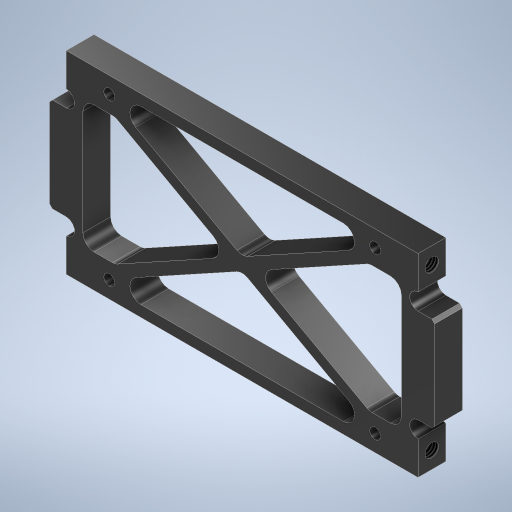
# Autodesk Inventor part: LegLinkBraceFrame
Saved by Autodesk Inventor 2024.2 (Build 282272000, 272)
## iProperties
Created: 2024-01-05
Part Number: LegLinkBraceFrame
Material: Aluminum 7075
Document SubType Name: Modeling
Designer: Masato Kubotera
Density: 2.81 g/cm^3
Appearance: Glossy - Black
Mass: 11.6625 g
Surface Area: 47.7408 cm^2
Volume: 4.15035 cm^3
Vendor: meviy
Author: Masato Kubotera
Autodesk Inventor part; units mm, degrees
ref_plane "YZ Plane" through (0, 0, 0) normal (1, 0, 0) x (0, 1, 0)
ref_plane "XZ Plane" through (0, 0, 0) normal (0, 1, 0) x (-1, 0, 0)
ref_plane "XY Plane" through (0, 0, 0) normal (0, 0, 1) x (1, 0, 0)
sketch "Sketch1" plane through (0, 0, 0) normal (1, 0, 0) x (0, 1, 0)
  line L0 (-31.75, 17.5) -> (31.75, 17.5)
  line L1 (31.75, 17.5) -> (31.75, -17.5)
  line L2 (31.75, -17.5) -> (-31.75, -17.5)
  line L3 (-31.75, -17.5) -> (-31.75, 17.5)
  line L4 (-31.75, 17.5) -> (31.75, -17.5) construction
  line L5 (31.75, 17.5) -> (-31.75, -17.5) construction
  line L6 (0, 17.5) -> (0, -17.5)
  line L7 (-31.75, 0) -> (31.75, 0) construction
  line L8 (31.75, 8.5) -> (34.75, 8.5)
  line L9 (34.75, 8.5) -> (34.75, -8.5)
  line L10 (34.75, -8.5) -> (31.75, -8.5)
  arc A0 (31.75, 11.5) -> (31.75, 8.5) centre (31.75, 10) ccw
  arc A1 (31.75, -8.5) -> (31.75, -11.5) centre (31.75, -10) ccw
  line L11 (31.75, 14.5) -> (25.75, 14.5) construction
  line L12 (26.75, 11.5) -> (23.4506, 11.5)
  line L13 (22.4852, 11.2516) -> (5.2495, 1.7516)
  line L14 (28.75, 9.5) -> (28.75, -9.5)
  line L15 (20.278, 13.5) -> (20.278, 13.5)
  line L16 (19.2434, 11.7484) -> (0.9654, 1.674)
  line L17 (18.278, 15.5) -> (-18.278, 15.5)
  line L18 (-20.278, 13.5) -> (-20.278, 13.5)
  line L19 (-19.2434, 11.7484) -> (-0.9654, 1.674)
  line L20 (26.75, -11.5) -> (23.4506, -11.5)
  line L21 (22.4852, -11.2516) -> (5.2495, -1.7516)
  arc A2 (20.278, 13.5) -> (18.278, 15.5) centre (18.278, 13.5) ccw
  arc A3 (19.2434, 11.7484) -> (20.278, 13.5) centre (18.278, 13.5) ccw
  arc A4 (-18.278, 15.5) -> (-20.278, 13.5) centre (-18.278, 13.5) ccw
  arc A5 (-20.278, 13.5) -> (-19.2434, 11.7484) centre (-18.278, 13.5) ccw
  arc A6 (-0.9654, 1.674) -> (0.9654, 1.674) centre (0, 3.4255) ccw
  arc A7 (23.4506, 11.5) -> (22.4852, 11.2516) centre (23.4506, 9.5) ccw
  arc A8 (28.75, 9.5) -> (26.75, 11.5) centre (26.75, 9.5) ccw
  arc A9 (26.75, -11.5) -> (28.75, -9.5) centre (26.75, -9.5) ccw
  arc A10 (22.4852, -11.2516) -> (23.4506, -11.5) centre (23.4506, -9.5) ccw
  arc A11 (5.2495, 1.7516) -> (5.2495, -1.7516) centre (6.2149, 0) ccw
  line L22 (25.75, 16) -> (25.75, 13) construction
  line L23 (19.2434, -11.7484) -> (0.9654, -1.674)
  line L24 (18.278, -15.5) -> (-18.278, -15.5)
  line L25 (-19.2434, -11.7484) -> (-0.9654, -1.674)
  arc A12 (18.278, -15.5) -> (20.278, -13.5) centre (18.278, -13.5) ccw
  arc A13 (20.278, -13.5) -> (19.2434, -11.7484) centre (18.278, -13.5) ccw
  arc A14 (-20.278, -13.5) -> (-18.278, -15.5) centre (-18.278, -13.5) ccw
  arc A15 (-19.2434, -11.7484) -> (-20.278, -13.5) centre (-18.278, -13.5) ccw
  arc A16 (0.9654, -1.674) -> (-0.9654, -1.674) centre (0, -3.4255) ccw
  line L26 (-26.75, 11.5) -> (-23.4506, 11.5)
  line L27 (-22.4852, 11.2516) -> (-5.2495, 1.7516)
  line L28 (-28.75, 9.5) -> (-28.75, -9.5)
  line L29 (-22.4852, -11.2516) -> (-5.2495, -1.7516)
  line L30 (-26.75, -11.5) -> (-23.4506, -11.5)
  arc A17 (-22.4852, 11.2516) -> (-23.4506, 11.5) centre (-23.4506, 9.5) ccw
  arc A18 (-26.75, 11.5) -> (-28.75, 9.5) centre (-26.75, 9.5) ccw
  arc A19 (-28.75, -9.5) -> (-26.75, -11.5) centre (-26.75, -9.5) ccw
  arc A20 (-23.4506, -11.5) -> (-22.4852, -11.2516) centre (-23.4506, -9.5) ccw
  arc A21 (-5.2495, -1.7516) -> (-5.2495, 1.7516) centre (-6.2149, 0) ccw
  line L31 (31.75, 0) -> (-31.75, 0) construction
  line L32 (-31.75, 8.5) -> (-34.75, 8.5)
  line L33 (-34.75, 8.5) -> (-34.75, -8.5)
  line L34 (-34.75, -8.5) -> (-31.75, -8.5)
  arc A22 (-31.75, 8.5) -> (-31.75, 11.5) centre (-31.75, 10) ccw
  arc A23 (-31.75, -11.5) -> (-31.75, -8.5) centre (-31.75, -10) ccw
  line L35 (31.75, -14.5) -> (25.75, -14.5) construction
  point P0 (0, 0)
  point P1 (22.9359, 11.5)
  point P2 (2.0716, 0)
  point P3 (20.278, 15.5)
  point P4 (20.278, 12.3187)
  point P5 (0, 1.1418)
  point P6 (-20.278, 15.5)
  point P7 (-20.278, 12.3187)
  point P8 (22.9359, -11.5)
  point P9 (-31.75, -11.5)
  point P10 (31.75, -11.5)
  point P11 (24, 14.5)
  point P12 (24, -14.5)
  point P13 (-24, 14.5)
  point P14 (-24, -14.5)
  dimension "d0" = 63.5
  dimension "d1" = 35
  dimension "d2" = 1.5
  dimension "d3" = 6
  dimension "d4" = 3
  dimension "d5" = 6
  dimension "d6" = 2
  dimension "d7" = 2
  dimension "d9" = 2
  dimension "d10" = 3
  dimension "d11" = 3
  dimension "d24" = 48
  constraints: 72 end point, 51 symmetric about line, 48 point on circle, 25 point on line, 24 centre point, 20 tangent, 9 equal radius, 7 midpoint, 6 horizontal, 4 parallel, 4 vertical, 2 coincident, 1 perpendicular, 16 other
  measures "d0" distance of L1.end L2.end
  measures "d1" distance of L0.end L1.end
  measures "d2" radius of A0
  measures "d3" distance of A0.start L0.end
  measures "d4" distance of L8.start L8.end
  measures "d5" distance of L11.end L11.start
  measures "d6" distance between parallel lines of L17 L0
  measures "d7" radius of A2
  measures "d9" distance between parallel lines of L13 L16
  measures "d10" distance between parallel lines of L1 L14
  measures "d11" distance of L22.start L22.end
  measures "d24" distance of point (-24, 14.5) point (24, 14.5)
extrude "Extrusion1" add sketch "Sketch1" along normal blind 5 contours L0 L6 L17 A4 A5 L19 A6 A16 L25 A15 A14 L24 L2 L3 A23 A22 | L0 L1 A0 A1 L2 L6 L24 A12 A13 L23 A16 A6 L16 A3 A2 L17 | L3 L34 L33 L32 | L8 L9 L10 L1
sketch "Sketch2" plane through (0, 31.75, 17.5) normal (0, 1, 0) x (1, 0, 0)
  line L0 (0, 6) -> (0, 0) projected
  line L1 (0, 3) -> (5, 3) construction
  line L2 (5, 6) -> (5, 0) projected
  line L3 (0, 35) -> (0, 29) projected
  line L4 (0, 32) -> (5, 32) construction
  line L5 (5, 35) -> (5, 29) projected
  point P0 (0, 17.5)
  point P1 (2.5, 32)
  point P2 (2.5, 3)
  constraints: 6 midpoint, 4 end point
hole "Hole1" at (2.5, 31.75, 14.5) at (2.5, 31.75, -14.5) direction (0, -1, 0) diameter 2.459 depth 6 thread size "M3x0.5" class "6H" standard "ANSI Metric M Profile"
mirror "Mirror1" about plane through (0, 0, 0) normal (0, 1, 0) of "Hole1"
chamfer "Chamfer1" distance 0.5 angle 45 4 edges at (2.5, 34.75, 8.5) (2.5, 34.75, -8.5) (2.5, -34.75, 8.5) (2.5, -34.75, -8.5)
hole "Hole2" at (0, 24, 14.5) at (0, 24, -14.5) at (0, -24, -14.5) at (0, -24, 14.5) direction (1, 0, 0) diameter 2 end through all
body "Solid1"
